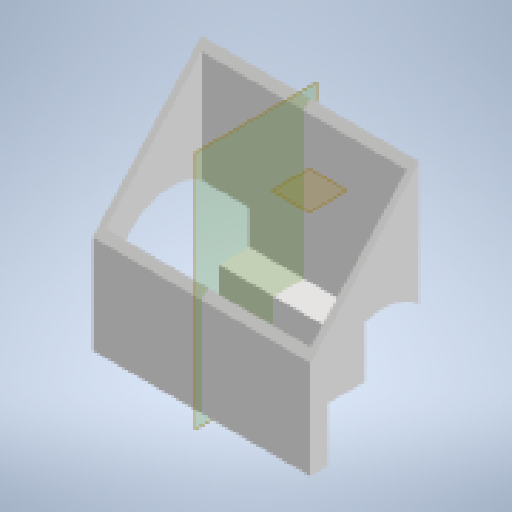
# Autodesk Inventor part: Shell
Saved by Autodesk Inventor 2025.1 (Build 291241020, 241B)
## iProperties
Created: 2025-01-12
Part Number: Shell
Material: Generic
Document SubType Name: Modeling
Designer: herme
Density: 1 g/cm^3
Appearance: Default
Author: herme
Autodesk Inventor part; units mm, degrees
ref_plane "YZ Plane" through (0, 0, 0) normal (1, 0, 0) x (0, 1, 0)
ref_plane "XZ Plane" through (0, 0, 0) normal (0, 1, 0) x (-1, 0, 0)
ref_plane "XY Plane" through (0, 0, 0) normal (0, 0, 1) x (1, 0, 0)
sketch "Sketch1" plane through (0, 0, 0) normal (0, 0, 1) x (1, 0, 0)
  line L0 (0, 0) -> (-100, 0)
  line L1 (-100, 0) -> (-100, -100)
  line L2 (-100, -100) -> (0, -100)
  line L3 (0, -100) -> (0, 0)
  dimension "d0" = 100
  dimension "d1" = 100
  constraints: 8 end point, 2 parallel, 1 horizontal, 1 perpendicular
  measures "d0" distance of L2.end L1.end
  measures "d1" distance of L1.end L0.end
extrude "Extrusion1" add sketch "Sketch1" along normal blind 50
shell "Shell1" thickness 3 removed faces 0
sketch "Sketch2" plane through (-100, -100, 0) normal (-1, 0, 0) x (0, 0, 1)
  circle A0 centre (17, 25) radius 25
  line L0 (0, 0) -> (50, 0) projected
  line L1 (0, 100) -> (0, 0) projected
  line L2 (42, 25) -> (42, 0)
  point P0 (0, 6.6697)
  dimension "d5" = 50
  dimension "d6" = 25
  dimension "d7" = 17
  constraints: 2 end point, 1 perpendicular, 1 point on line, 3 other
  measures "d6" distance from line of L0 point (17, 25)
  measures "d7" distance from line of L1 point (17, 25)
extrude "Wheel Hole" cut sketch "Sketch2" against normal blind 25
ref_plane "Mirror Plane" through (-50, -100, 50) normal (-1, 0, 0) x (0, 0, 1)
mirror "Mirror Wheel" about plane through (-50, -100, 50) normal (-1, 0, 0) of "Wheel Hole"
sketch "Sketch4" plane through (-100, -100, 50) normal (0, -1, 0) x (1, 0, 0)
  line L0 (25, -8) -> (25, -50) projected
  line L1 (25, -50) -> (75, -50)
  line L2 (75, -50) -> (75, -33)
  line L3 (75, -33) -> (25, -33)
  line L4 (25, -33) -> (25, -50)
  line L5 (25, -50) -> (75, -50) projected
  point P0 (100, -50)
  dimension "d11" = 17
  dimension "d13" = 17
  constraints: 8 end point, 2 parallel, 1 horizontal, 1 perpendicular, 1 point on line
  measures "d11" distance of L2.end L1.end
  measures "d13" distance between parallel lines of L5 L3
extrude "Motor Stand" add sketch "Sketch4" against normal blind 30
sketch "Sketch5" plane through (-100, -100, 50) normal (-1, 0, 0) x (0, 0, 1)
  line L0 (-50, 100) -> (0, 45)
  line L1 (0, 100) -> (0, 0) projected
  line L2 (-8, 0) -> (0, 0) projected
  line L3 (-50, 100) -> (0, 100) projected
  line L4 (-50, 100) -> (0, 100)
  line L5 (0, 100) -> (0, 45)
  point P0 (-4, 0)
  dimension "d16" = 45
  constraints: 6 end point, 1 collinear, 1 midpoint, 1 perpendicular, 1 point on line
  measures "d16" vertical distance of point (-4, 0) L0.end
extrude "Ramp Cut" cut sketch "Sketch5" against normal through all
sketch "Sketch9" plane through (-100, -100, 42) normal (-1, 0, 0) x (0, 0, 1)
  line L0 (-39, 45.7123) -> (-39, 96.7) projected
  line L1 (-39, 93.7) -> (5, 45.3)
  line L2 (5, 3) -> (5, 48.3) projected
  line L3 (8, 45) -> (-42, 100) projected
  dimension "d44" = 3
  dimension "d45" = 3
  constraints: 2 end point, 2 point on line
  measures "d44" distance of L0.end L1.start
  measures "d45" distance of L2.end L1.end
extrude "Ramp Cover" add sketch "Sketch9" against normal through all
sketch "Sketch6" plane through (-100, -100, 50) normal (0, -1, 0) x (1, 0, 0)
  line L0 (38.75, -8) -> (43.75, -8)
  line L1 (43.75, -8) -> (43.75, -33)
  line L2 (43.75, -33) -> (38.75, -33)
  line L3 (38.75, -33) -> (38.75, -8)
  line L4 (56.25, -8) -> (61.25, -8)
  line L5 (61.25, -8) -> (61.25, -33)
  line L6 (61.25, -33) -> (56.25, -33)
  line L7 (56.25, -33) -> (56.25, -8)
  line L8 (43.75, -18.5) -> (56.25, -18.5)
  line L9 (56.25, -18.5) -> (56.25, -22.5)
  line L10 (56.25, -22.5) -> (43.75, -22.5)
  line L11 (43.75, -22.5) -> (43.75, -18.5)
  line L12 (0, 0) -> (100, 0) projected
  line L13 (25, -8) -> (25, -50) projected
  point P0 (100, -50)
  point P1 (43.75, -20.5)
  point P2 (38.75, -20.5)
  dimension "d19" = 5
  dimension "d20" = 25
  dimension "d21" = 5
  dimension "d22" = 25
  dimension "d23" = 12.5
  dimension "d24" = 4
  dimension "d25" = 8
  dimension "d26" = 0
  dimension "d27" = 0
  dimension "d28" = 10.5
  dimension "d29" = 13.75
  constraints: 24 end point, 6 parallel, 3 horizontal, 3 perpendicular, 2 midpoint, 1 point on line
  measures "d19" distance of L1.end L2.end
  measures "d20" distance of L0.end L1.end
  measures "d21" distance of L5.end L6.end
  measures "d22" distance of L4.end L5.end
  measures "d23" distance of L9.end L10.end
  measures "d24" distance of L8.end L9.end
  measures "d25" distance between parallel lines of L12 L0
  measures "d26" distance from line of point (43.75, -20.5) L1
  measures "d27" distance between parallel lines of L7 L9
  measures "d28" distance between parallel lines of L4 L8
  measures "d29" distance from line of L13 point (38.75, -20.5)
extrude "H Logo" cut sketch "Sketch6" against normal up to surface (3 mm away)
ref_plane "Peephole Plane" through (-50, -23.8, 13) normal (0, 1, 0) x (1, 0, 0)
sketch "Sketch7" plane through (-50, -23.8, 13) normal (0, 1, 0) x (1, 0, 0)
  circle A0 centre (12.5, 0) radius 8.5
  line L0 (47, -34) -> (47, 10) projected
  line L1 (47, 10) -> (-47, 10) projected
  circle A1 centre (-12.5, 0) radius 8.5
  line L2 (6.25, -4) -> (-6.25, -4) projected
  arc A2 (-6.5, 6.0208) -> (6.5, 6.0208) centre (0, 12.5433) ccw
  arc A3 (6.5, -6.0208) -> (-6.5, -6.0208) centre (0, -12.5429) ccw
  point P0 (50, 13)
  point P1 (0, -3.3349)
  point P2 (-3.4361, -4)
  point P3 (3.4361, -4)
  point P4 (5, -4)
  point P5 (-5, -4)
  dimension "d32" = 17
  dimension "d33" = 34.5
  dimension "d34" = 10
  dimension "d38" = 25
  dimension "d62" = 6
  dimension "d63" = 6
  dimension "d64" = 6
  dimension "d65" = 6
  dimension "d67" = 9.208
  constraints: 9 point on circle, 4 centre point, 1 horizontal, 1 tangent, 2 other
  measures "d32" diameter of A0
  measures "d33" distance from line of L0 A0.centre
  measures "d34" distance from line of L1 A0.centre
  measures "d38" distance of A0.centre A1.centre
  measures "d62" horizontal distance of A0.centre A0.start
  measures "d63" horizontal distance of A1.centre A1.start
  measures "d64" horizontal distance of A0.centre A0.end
  measures "d65" horizontal distance of A1.centre A1.end
  measures "d67" radius of A3
extrude "Peephole" cut sketch "Sketch7" along normal through all contours A0 | A0 L2 A3 A1 A2 | A3 L2 A0 | A1 | A1 L2 A3
sketch "Sketch17" plane through (-100, 0, 0) normal (0, 0.6726728, 0.7399401) x (1, 0, 0)
  line L0 (60.2513, -62.008) -> (63.7868, -65.5435)
  line L1 (63.7868, -65.5435) -> (85, -44.3303)
  line L2 (85, -44.3303) -> (81.4645, -40.7948)
  line L3 (81.4645, -40.7948) -> (60.2513, -62.008)
  line L4 (60.2513, -62.008) -> (65.2513, -62.008) construction
  line L5 (85, -62.008) -> (81.4645, -65.5435)
  line L6 (81.4645, -65.5435) -> (60.2513, -44.3303)
  line L7 (60.2513, -44.3303) -> (63.7868, -40.7948)
  line L8 (63.7868, -40.7948) -> (85, -62.008)
  line L9 (85, -62.008) -> (90, -62.008) construction
  line L10 (100, 0) -> (100, -74.3303) projected
  line L11 (100, -74.3303) -> (0, -74.3303) projected
  line L12 (39.75, -62.008) -> (36.2145, -65.5435)
  line L13 (18.5368, -40.7948) -> (39.75, -62.008)
  line L14 (36.2145, -65.5435) -> (15.0013, -44.3303)
  line L15 (15.0013, -44.3303) -> (18.5368, -40.7948)
  line L16 (36.2145, -40.7948) -> (15.0013, -62.008)
  line L17 (39.75, -44.3303) -> (36.2145, -40.7948)
  line L18 (18.5368, -65.5435) -> (39.75, -44.3303)
  line L19 (15.0013, -62.008) -> (18.5368, -65.5435)
  point P0 (27.3756, -56.7047)
  point P1 (30.9112, -53.1692)
  point P2 (27.3756, -49.6336)
  point P3 (23.8401, -53.1692)
  point P4 (72.6256, -49.6336)
  point P5 (69.0901, -53.1692)
  point P6 (72.6256, -56.7047)
  point P7 (76.1612, -53.1692)
  dimension "d82" = 5
  dimension "d83" = 45
  dimension "d84" = 30
  dimension "d85" = 5
  dimension "d86" = 135
  dimension "d87" = 30
  dimension "d88" = 15
  dimension "d89" = 30
  dimension "d92" = 15
  dimension "d93" = 30
  dimension "d96" = 45.25
  constraints: 36 end point, 4 parallel, 3 horizontal, 2 equal length, 2 perpendicular, 16 other
  measures "d82" distance of L0.start L0.end
  measures "d83" angle of L0 L4
  measures "d84" distance of L1.end L0.end
  measures "d85" distance of L5.start L5.end
  measures "d86" angle of L5 L9
  measures "d87" distance of L5.end L6.end
  measures "d88" distance from line of L10 L1.end
  measures "d89" distance from line of L11 L1.end
  measures "d92" distance from line of L10 L5.start
  measures "d93" distance from line of L11 L6.end
  measures "d96" distance of L5.start L12.start
extrude "Exes" cut sketch "Sketch17" against normal up to surface (2.018 mm away)
sketch "Sketch19" plane through (-97, -54.2877, 3) normal (0, 0, 1) x (1, 0, 0)
  line L0 (52, 43.9877) -> (42, 43.9877)
  line L1 (42, 43.9877) -> (42, 33.9877)
  line L2 (42, 33.9877) -> (52, 33.9877)
  line L3 (52, 33.9877) -> (52, 43.9877)
  line L4 (94, 50.9877) -> (0, 50.9877) projected
  line L5 (94, 2.5877) -> (94, 50.9877) projected
  line L6 (52, 1.9877) -> (52, 11.9877)
  line L7 (52, 11.9877) -> (42, 11.9877)
  line L8 (42, 11.9877) -> (42, 1.9877)
  line L9 (42, 1.9877) -> (52, 1.9877)
  point P0 (97, 54.2877)
  dimension "d105" = 10
  dimension "d106" = 10
  dimension "d107" = 7
  dimension "d108" = 42
  dimension "d111" = 32
  constraints: 16 end point, 2 parallel, 1 horizontal, 1 perpendicular, 1 vertical, 8 other
  measures "d105" distance of L2.end L1.end
  measures "d106" distance of L1.end L0.end
  measures "d107" distance between parallel lines of L4 L0
  measures "d108" distance between parallel lines of L5 L3
  measures "d111" distance of L2.end L6.start
extrude "Extrusion15" cut sketch "Sketch19" against normal blind 10
chamfer "Chamfer1" distance 3 angle 45 12 edges at (-61.25, -100, 29.5) (-56.25, -100, 36.75) (-56.25, -100, 22.25) (-58.75, -100, 17) (-58.75, -100, 42) (-50, -100, 31.5) (-50, -100, 27.5) (-43.75, -100, 36.75) (-41.25, -100, 42) (-38.75, -100, 29.5) (-41.25, -100, 17) (-43.75, -100, 22.25)
body "Solid1"
